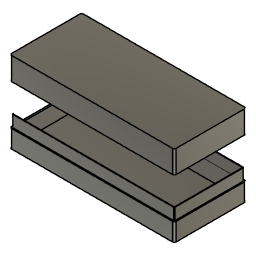
saw_box v1 (Autodesk Fusion 360 design; units mm, degrees)
Autodesk Fusion 360 part; units mm, degrees
note: some values were not read from the file. Chosen so that the rebuilt part matches the saved one: which bodies a step acts on; which face or edge a step refers to.
sketch "草图1" plane through (0, 0, 0) normal (0, 0, 1) x (1, 0, 0)
  line L0 (0, 0) -> (280, 0)
  line L1 (280, 0) -> (280, 120)
  line L2 (280, 120) -> (0, 120)
  line L3 (0, 120) -> (0, 0)
  line L4 (-2, 122) -> (282, 122)
  line L5 (282, 122) -> (282, -2)
  line L6 (282, -2) -> (-2, -2)
  line L7 (-2, -2) -> (-2, 122)
  dimension "d1" = 280
  dimension "d2" = 120
  dimension "d3" = 2
  dimension "d4" = 2
  dimension "d5" = 2
  dimension "d6" = 2
  constraint horizontal L0
  constraint vertical L1
  constraint horizontal L2
  constraint vertical L3
  constraint coincident L0.start L3.end
  constraint horizontal L4
  constraint vertical L5
  constraint horizontal L6
  constraint vertical L7
  measures "d1" distance of L1 L3
  measures "d2" distance of L0 L2
  measures "d3" distance of L2 L4
  measures "d4" distance of L3 L7
  measures "d5" distance of L1 L5
  measures "d6" distance of L0 L6
extrude "拉伸1" add sketch "草图1" along normal blind 70 contours L0 L1 L2 L3 | L4 L5 L6 L7 makes body 1
sketch "草图2" plane through (0, -2, 0) normal (0, -1, 0) x (1, 0, 0)
  line L0 (-2, 0) -> (282, 0)
  line L1 (282, 0) -> (282, 70)
  line L2 (282, 70) -> (-2, 70)
  line L3 (-2, 70) -> (-2, 0)
  line L4 (-2, 50.8835) -> (282, 50.8835)
  constraint coincident L3 L4.start
  constraint coincident L1 L4.end
  constraint perpendicular L1 L4
split "分割1" by curves path "草图2" along L4 bodies 1 makes body 2 at (92.6667, 80.6667, 0)
move_body "移动1" bodies 1 to x (1, 0, 0) y (0, 1, 0) z (0, 0, 1) at (0, 0, 100)
shell "抽壳1" thickness 3 removed faces 1 at (92.6667, 39.3333, 50.8835) on bodies 2
shell "抽壳2" thickness 3 removed faces 1 at (92.6667, 39.3333, 150.8835) on bodies 1
fillet "圆角1" radius 3 8 edges at (282, -2, 160.4417) (-2, -2, 160.4417) (-2, 122, 160.4417) (282, 122, 160.4417) (-2, -2, 25.4417) (282, -2, 25.4417) (-2, 122, 25.4417) (282, 122, 25.4417) on bodies 1 2
sketch "草图3" plane through (0, 0, 50.8835) normal (0, 0, 1) x (-1, 0, 0)
  line L0 (-279, -119) -> (-279, -1)
  line L1 (-279, -1) -> (-1, -1)
  line L2 (-1, -1) -> (-1, -119)
  line L3 (-1, -119) -> (-279, -119)
  arc A0 (-282, -119) -> (-279, -122) centre (-279, -119) ccw
  line L4 (-279, -122) -> (-1, -122)
  arc A1 (-1, -122) -> (2, -119) centre (-1, -119) ccw
  line L5 (2, -119) -> (2, -1)
  arc A2 (2, -1) -> (-1, 2) centre (-1, -1) ccw
  line L6 (-1, 2) -> (-279, 2)
  arc A3 (-279, 2) -> (-282, -1) centre (-279, -1) ccw
  line L7 (-282, -1) -> (-282, -119)
  line L8 (-279, 0) -> (-1, 0)
  line L9 (0, -1.5) -> (0, -119.1588)
  line L10 (-1, -120) -> (-279, -120)
  line L11 (-280, -119) -> (-280, -1)
  circle A4 centre (-1, -119) radius 1
  circle A5 centre (-1, -1) radius 1
  circle A6 centre (-279, -1) radius 1
  circle A7 centre (-279, -119) radius 1
  dimension "d13" = 1
  dimension "d14" = 1
  dimension "d15" = 1
  dimension "d16" = 1
  dimension "d17" = 1
  dimension "d18" = 1
  dimension "d19" = 1
  dimension "d20" = 1
  constraint perpendicular L2 L8
  constraint perpendicular L8 L9
  constraint perpendicular L2 L10
  constraint perpendicular L3 L11
  constraint tangent L9 A4
  constraint tangent L10 A4
  constraint tangent L8 A5
  constraint tangent L9 A5
  constraint tangent L8 A6
  constraint tangent L11 A6
  constraint tangent L11 A7
  constraint tangent L10 A7
  measures "d13" distance of L0 L11
  measures "d14" distance of L1 L8
  measures "d15" distance of L2 L9
  measures "d16" distance of L3 L10
  measures "d17" radius of A4
  measures "d18" radius of A5
  measures "d19" radius of A6
  measures "d20" radius of A7
extrude "拉伸2" cut sketch "草图3" against normal blind 20 bodies 2
move_body "移动2" bodies 1 to x (1, 0, 0) y (0, 1, 0) z (0, 0, 1) at (0, 0, -100)
extrude "拉伸4" add sketch "草图3" against normal blind 20 bodies 1
move_body "移动3" bodies 1 to x (1, 0, 0) y (0, 1, 0) z (0, 0, 1) at (0, 0, 70)
